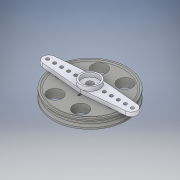
# Autodesk Inventor part: servo-roller-wheel-attachment
Saved by Autodesk Inventor 2019 (Build 230136000, 136)
## iProperties
Created: 2019-04-14
Part Number: servo-roller-wheel-attachment
Material: Generic
Document SubType Name: Modeling
Designer: Tesler
Density: 1 g/cm^3
Appearance: Default
Author: Tesler
Autodesk Inventor part; units mm, degrees
ref_plane "YZ Plane" through (0, 0, 0) normal (1, 0, 0) x (0, 1, 0)
ref_plane "XZ Plane" through (0, 0, 0) normal (0, 1, 0) x (-1, 0, 0)
sketch "Sketch1" plane through (0, 0, 0) normal (0, 1, 0) x (-1, 0, 0)
  circle A0 centre (0, 0) radius 11.5
  circle A1 centre (8, 0) radius 2.25
  circle A2 centre (4, 6.928203) radius 2.25
  circle A3 centre (-4, 6.928203) radius 2.25
  circle A4 centre (-8, 0) radius 2.25
  circle A5 centre (-4, -6.928203) radius 2.25
  circle A6 centre (4, -6.928203) radius 2.25
  dimension "d0" = 23
  dimension "d1" = 4.5
  dimension "d2" = 8
  dimension "d5" = 360
  constraints: 7 centre point, 1 coincident, 13 other
  measures "d0" diameter of A0
  measures "d1" diameter of A1
  measures "d2" distance of point (0, 0) A1.centre
extrude "Extrusion1" add sketch "Sketch1" along normal blind 3
ref_plane "Work Plane1" through (0, 1.5, 0) normal (0, 1, 0) x (1, 0, 0)
sketch "Sketch2" plane through (0, 1.5, 0) normal (0, 1, 0) x (1, 0, 0)
  circle A0 centre (0, 0) radius 11.5 projected
  circle A1 centre (0, 0) radius 11.5
  circle A2 centre (0, 0) radius 11
  dimension "d11" = 22
  constraints: 2 centre point, 2 coincident, 1 concentric
  measures "d11" diameter of A2
extrude "Extrusion2" cut sketch "Sketch2" along normal mid plane 2
fillet "Fillet1" radius 0.7 2 edges at (-11, 2.5, 0) (-11, 0.5, 0)
sketch "Sketch3" plane through (0, 3, 0) normal (0, 1, 0) x (1, 0, 0)
  arc A0 (-12.996246, 1.823729) -> (-12.996246, -1.823729) centre (-12.831183, 0) ccw
  circle A1 centre (0, 0) radius 11
  line L0 (0, -3) -> (-12.996246, -1.823729)
  line L1 (0, 3) -> (-12.996246, 1.823729)
  line L2 (0, 16.1) -> (0, -16.1)
  arc A2 (12.996246, -1.823729) -> (12.996246, 1.823729) centre (12.831183, 0) ccw
  line L3 (0, -3) -> (12.996246, -1.823729)
  line L4 (0, 3) -> (12.996246, 1.823729)
  arc A3 (0.538639, 2.951249) -> (-0.538639, 2.951249) centre (0, 0) ccw
  arc A4 (-0.538639, -2.951249) -> (0.538639, -2.951249) centre (0, 0) ccw
  dimension "d14" = 3.66237
  dimension "d15" = 10.3433
  dimension "d16" = 25.66237
  dimension "d17" = 10.3433
  dimension "d18" = 6
  dimension "d19" = 2.98779
  constraints: 10 point on circle, 8 end point, 4 centre point, 4 point on line, 3 symmetric about line, 3 tangent, 1 coincident, 1 other
  measures "d14" diameter of A0
  measures "d15" angle of L1 L0
  measures "d16" distance of A0.centre A2.centre
  measures "d17" angle of L4 L3
  measures "d18" distance of L1.start L0.start
  measures "d19" distance from line of point (0, 0) L3
extrude "Extrusion3" add sketch "Sketch3" along normal blind 1.25 contours L1 A1 L0 A0 | L1 L2 L0 A1 | L4 A2 L3 A1 | A1 L3 L2 L4
sketch "Sketch8" plane through (0, 3, 0) normal (0, 1, 0) x (1, 0, 0)
  arc A0 (-11.329206, -1.97461) -> (11.329206, -1.97461) centre (0, 0) ccw
  circle A1 centre (0, 0) radius 11
  dimension "d65" = 22
  constraints: 1 centre point, 1 coincident
  measures "d65" diameter of A1
extrude "Extrusion8" cut sketch "Sketch8" against normal blind 0.2
sketch "Sketch4" plane through (0, 4.25, 0) normal (0, 1, 0) x (1, 0, 0)
  line L0 (0, 3) -> (11.329206, 1.97461)
  circle A0 centre (0, 0) radius 3
  circle A1 centre (0, 0) radius 2.5
  dimension "d22" = 5
  constraints: 2 coincident, 1 centre point, 1 vertical alignment, 2 other
  measures "d22" diameter of A1
extrude "Extrusion4" add sketch "Sketch4" along normal blind 1.25
sketch "Sketch9" plane through (0, 0, 0) normal (0, -1, 0) x (1, 0, 0)
  circle A0 centre (0, 0) radius 11
  dimension "d68" = 22
  constraints: 1 centre point, 1 coincident
  measures "d68" diameter of A0
extrude "Extrusion9" cut sketch "Sketch9" against normal blind 0.2
sketch "Sketch5" plane through (0, 0, 0) normal (0, -1, 0) x (1, 0, 0)
  circle A0 centre (0, 0) radius 2.5
  dimension "d25" = 5
  constraints: 1 centre point, 1 coincident
  measures "d25" diameter of A0
extrude "Extrusion5" add sketch "Sketch5" along normal blind 0.5 and the other way blind 0.25
sketch "Sketch6" plane through (0, -0.5, 0) normal (0, -1, 0) x (1, 0, 0)
  circle A0 centre (0, 0) radius 2.5
  arc A1 (-0.25, -3.5) -> (0.25, -3.5) centre (0, -3.5) ccw
  line L0 (-0.25, -3.5) -> (-0.25, -2.25)
  line L1 (0.25, -3.5) -> (0.25, -2.243733)
  arc A2 (-0.4, -2.25) -> (-2.186134, -0.532276) centre (-2.149709, -2.281897) ccw
  line L2 (0, -16.1) -> (0, 16.1)
  arc A3 (2.184345, -0.539571) -> (0.4, -2.25) centre (2.14956, -2.289225) ccw
  line L3 (-0.25, -2.25) -> (-0.4, -2.25)
  line L4 (0.25, -2.25) -> (0.4, -2.25)
  line L5 (-20.527313, 0) -> (20.527313, 0)
  arc A4 (0.25, 3.5) -> (-0.25, 3.5) centre (0, 3.5) ccw
  line L6 (-0.25, 3.5) -> (-0.25, 2.25)
  line L7 (0.25, 3.5) -> (0.25, 2.243733)
  arc A5 (-2.186134, 0.532276) -> (-0.4, 2.25) centre (-2.149709, 2.281897) ccw
  arc A6 (0.4, 2.25) -> (2.184345, 0.539571) centre (2.14956, 2.289225) ccw
  line L8 (-0.25, 2.25) -> (-0.4, 2.25)
  line L9 (0.25, 2.25) -> (0.4, 2.25)
  arc A7 (-2.186134, 0.532276) -> (-2.186134, -0.532276) centre (0, 0) ccw
  arc A8 (2.184345, -0.539571) -> (2.184345, 0.539571) centre (0, 0) ccw
  point P0 (0, -2.25)
  point P1 (-2.25, 0)
  point P2 (2.184345, -0.539571)
  point P3 (2.25, 0)
  dimension "d28" = 3.5
  dimension "d29" = 0.5
  dimension "d34" = 1.75
  dimension "d35" = 1.75
  dimension "d37" = 2.25
  dimension "d38" = 4.5
  dimension "d39" = 4.5
  dimension "d40" = 7
  dimension "d41" = 0.5
  dimension "d42" = 4.37048
  dimension "d43" = 2.96772
  dimension "d44" = 1.78435
  dimension "d45" = 1.78613
  dimension "d46" = 1.71043
  dimension "d47" = 27.368
  dimension "d48" = 76.125
  dimension "d49" = 2.25
  constraints: 18 point on circle, 16 end point, 12 symmetric about line, 8 centre point, 2 horizontal, 2 point on line, 2 vertical, 1 coincident, 3 other
  measures "d28" distance of A0.centre point (0, -3.5)
  measures "d29" diameter of A1
  measures "d34" radius of A2
  measures "d35" radius of A3
  measures "d37" radius of A7
  measures "d38" distance between parallel lines of L8 L3
  measures "d39" distance between parallel lines of L9 L4
  measures "d40" distance of A4.centre point (0, -3.5)
  measures "d41" distance between parallel lines of L0 L1
  measures "d42" distance of point (2.184, -0.54) A2.end
  measures "d43" vertical distance of A2.end A1.centre
  measures "d44" horizontal distance of A3.start L4.end
  measures "d45" horizontal distance of L8.end A5.start
  measures "d46" vertical distance of A6.end L9.end
  measures "d49" radius of A8
extrude "Extrusion6" cut sketch "Sketch6" against normal blind 3.5 contours L7 L9 A6 A8 L5 L2 A0 | A0 L2 A4 L7 | L1 A1 L2 A0 | A0 L2 L5 A8 A3 L4 L1 | L2 L5 A7 A5 L8 L6 A0 | A0 L6 A4 L2 | L2 A1 L0 A0 | A0 L0 L3 A2 A7 L5 L2
sketch "Sketch7" plane through (0, 4.25, 0) normal (0, 1, 0) x (1, 0, 0)
  arc A0 (-0.538639, 2.951249) -> (-0.538639, -2.951249) centre (0, 0) ccw
  line L0 (-0.538639, 2.951249) -> (-12.996246, 1.823729)
  arc A1 (-12.996246, 1.823729) -> (-12.996246, -1.823729) centre (-12.831183, 0) ccw
  line L1 (-12.996246, -1.823729) -> (-0.538639, -2.951249)
  arc A2 (-12.996246, 1.823729) -> (-12.996246, -1.823729) centre (-12.831183, 0) ccw
  circle A3 centre (-13.204571, 0) radius 0.5
  circle A4 centre (-11.017877, 0) radius 0.5
  circle A5 centre (-8.831183, 0) radius 0.5
  circle A6 centre (-6.644489, 0) radius 0.5
  circle A7 centre (-4.457796, 0) radius 0.5
  line L2 (0, 16.1) -> (0, -16.1)
  circle A8 centre (13.204571, 0) radius 0.5
  circle A9 centre (11.017877, 0) radius 0.5
  circle A10 centre (8.831183, 0) radius 0.5
  circle A11 centre (6.644489, 0) radius 0.5
  circle A12 centre (4.457796, 0) radius 0.5
  circle A13 centre (0, 0) radius 1.000558
  point P0 (-3, 0)
  point P1 (-14.662366, 0)
  dimension "d52" = 11.66237
  dimension "d53" = 1.4578
  dimension "d54" = 3.64449
  dimension "d55" = 8.01788
  dimension "d56" = 10.20457
  dimension "d57" = 5.83118
  dimension "d58" = 1
  dimension "d59" = 1
  dimension "d60" = 1
  dimension "d61" = 1
  dimension "d62" = 1
  dimension "d74" = 2.00112
  constraints: 11 centre point, 6 coincident, 5 symmetric about line, 3 point on circle, 5 other
  measures "d52" distance of point (-3, 0) point (-14.662, 0)
  measures "d53" distance of point (-14.662, 0) point (-13.205, 0)
  measures "d54" distance of point (-11.018, 0) point (-14.662, 0)
  measures "d55" distance of point (-6.644, 0) point (-14.662, 0)
  measures "d56" distance of point (-4.458, 0) point (-14.662, 0)
  measures "d57" distance of point (-8.831, 0) point (-14.662, 0)
  measures "d58" diameter of A3
  measures "d59" diameter of A4
  measures "d60" diameter of A5
  measures "d61" diameter of A6
  measures "d62" diameter of A7
  measures "d74" diameter of A13
extrude "Extrusion7" cut sketch "Sketch7" against normal blind 1.25 contours A3 | A4 | A5 | A6 | A7 | A13 L2 | L2 A13 | A8 | A9 | A10 | A11 | A12
fillet "Fillet2" radius 0.7 2 edges at (-11, 2.8, 0) (-11, 0.2, 0)
sketch "Sketch10" plane through (0, 0.2, 0) normal (0, -1, 0) x (1, 0, 0)
  circle A0 centre (8, 0) radius 2.25
  circle A1 centre (-8, 0) radius 2.25
  circle A2 centre (8, 0) radius 2.25
  circle A3 centre (-8, 0) radius 2.266667
  line L0 (-0.538639, -2.951249) -> (-12.996246, -1.823729)
  point P0 (0, 0)
  constraints: 2 centre point, 2 coincident, 1 concentric, 1 tangent
sketch "Sketch10 outline for Extrusion10" plane through (0, 0.2, 0) normal (0, -1, 0) x (1, 0, 0)
  circle A0 centre (8, 0) radius 2.25
  circle A1 centre (-8, 0) radius 2.25
extrude "Extrusion10" add sketch "Sketch10 outline for Extrusion10" against normal blind 2.8 and the other way blind 0.1
sketch "Sketch11" plane through (-8, 0.1, 0) normal (0, -1, 0) x (1, 0, 0)
  circle A0 centre (16, 0) radius 2.25 projected
  circle A1 centre (0, 0) radius 2.25 projected
  circle A2 centre (0, 0) radius 2
  circle A3 centre (16, 0) radius 2
  point P0 (8, 0)
  dimension "d79" = 4
  dimension "d80" = 4
  constraints: 2 centre point, 2 coincident
  measures "d79" diameter of A2
  measures "d80" diameter of A3
extrude "Extrusion11" add sketch "Sketch11" along normal blind 0.2 contours A2 | A3
fillet "Fillet3" radius 0.7 2 edges at (-10, -0.1, 0) (6, -0.1, 0)
equation "\"d53\" = 0.125 * d52"
equation "\"d54\" = 2.5 * d53"
equation "\"d55\" = 5.5 * d53"
equation "\"d56\" = 7 * d53"
equation "\"d57\" = 4 * d53"
body "Solid1"
